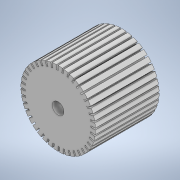
# Autodesk Inventor part: gear(1.5 inch)
Saved by Autodesk Inventor 2022 (Build 260153000, 153)
## iProperties
Created: 2021-07-02
Part Number: gear(1.5 inch)
Material: Generic
Document SubType Name: Modeling
Designer: hp
Density: 1 g/cm^3
Appearance: Default
Author: hp
Autodesk Inventor part; units mm, degrees
ref_plane "YZ Plane" through (0, 0, 0) normal (1, 0, 0) x (0, 1, 0)
ref_plane "XZ Plane" through (0, 0, 0) normal (0, 1, 0) x (-1, 0, 0)
ref_plane "XY Plane" through (0, 0, 0) normal (0, 0, 1) x (1, 0, 0)
sketch "Sketch1" plane through (0, 0, 0) normal (0, 0, 1) x (1, 0, 0)
  circle A0 centre (0, 0) radius 19.05
  dimension "d0" = 38.1
  constraints: 1 centre point, 1 coincident
  measures "d0" diameter of A0
extrude "Extrusion1" add sketch "Sketch1" along normal blind 32.639
sketch "Sketch2" plane through (0, 0, 32.639) normal (0, 0, 1) x (1, 0, 0)
  circle A0 centre (0, 0) radius 19.05 projected
  line L0 (-19.05, 0) -> (-16.815, 0)
  line L1 (-16.815, 0) -> (-16.815, -0.745)
  line L2 (-16.815, -0.745) -> (-19.05, -0.745)
  line L3 (-19.05, -0.745) -> (-19.05, 0)
  line L4 (-18.8155, -2.9801) -> (-16.608, -2.6304)
  line L5 (-16.608, -2.6304) -> (-16.4914, -3.3663)
  line L6 (-16.4914, -3.3663) -> (-18.6989, -3.7159)
  line L7 (-18.6989, -3.7159) -> (-18.8155, -2.9801)
  line L8 (-18.1176, -5.8868) -> (-15.992, -5.1961)
  line L9 (-15.992, -5.1961) -> (-15.7618, -5.9047)
  line L10 (-15.7618, -5.9047) -> (-17.8874, -6.5953)
  line L11 (-17.8874, -6.5953) -> (-18.1176, -5.8868)
  line L12 (-16.9737, -8.6485) -> (-14.9823, -7.6339)
  line L13 (-14.9823, -7.6339) -> (-14.6441, -8.2977)
  line L14 (-14.6441, -8.2977) -> (-16.6355, -9.3123)
  line L15 (-16.6355, -9.3123) -> (-16.9737, -8.6485)
  line L16 (-15.4118, -11.1973) -> (-13.6036, -9.8836)
  line L17 (-13.6036, -9.8836) -> (-13.1657, -10.4863)
  line L18 (-13.1657, -10.4863) -> (-14.9739, -11.8)
  line L19 (-14.9739, -11.8) -> (-15.4118, -11.1973)
  line L20 (-13.4704, -13.4704) -> (-11.89, -11.89)
  line L21 (-11.89, -11.89) -> (-11.3632, -12.4168)
  line L22 (-11.3632, -12.4168) -> (-12.9436, -13.9972)
  line L23 (-12.9436, -13.9972) -> (-13.4704, -13.4704)
  line L24 (-11.1973, -15.4118) -> (-9.8836, -13.6036)
  line L25 (-9.8836, -13.6036) -> (-9.2809, -14.0415)
  line L26 (-9.2809, -14.0415) -> (-10.5946, -15.8497)
  line L27 (-10.5946, -15.8497) -> (-11.1973, -15.4118)
  line L28 (-8.6485, -16.9737) -> (-7.6339, -14.9823)
  line L29 (-7.6339, -14.9823) -> (-6.9701, -15.3205)
  line L30 (-6.9701, -15.3205) -> (-7.9847, -17.3119)
  line L31 (-7.9847, -17.3119) -> (-8.6485, -16.9737)
  line L32 (-5.8868, -18.1176) -> (-5.1961, -15.992)
  line L33 (-5.1961, -15.992) -> (-4.4876, -16.2222)
  line L34 (-4.4876, -16.2222) -> (-5.1782, -18.3478)
  line L35 (-5.1782, -18.3478) -> (-5.8868, -18.1176)
  line L36 (-2.9801, -18.8155) -> (-2.6304, -16.608)
  line L37 (-2.6304, -16.608) -> (-1.8946, -16.7245)
  line L38 (-1.8946, -16.7245) -> (-2.2442, -18.932)
  line L39 (-2.2442, -18.932) -> (-2.9801, -18.8155)
  line L40 (0, -19.05) -> (0, -16.815)
  line L41 (0, -16.815) -> (0.745, -16.815)
  line L42 (0.745, -16.815) -> (0.745, -19.05)
  line L43 (0.745, -19.05) -> (0, -19.05)
  line L44 (2.9801, -18.8155) -> (2.6304, -16.608)
  line L45 (2.6304, -16.608) -> (3.3663, -16.4914)
  line L46 (3.3663, -16.4914) -> (3.7159, -18.6989)
  line L47 (3.7159, -18.6989) -> (2.9801, -18.8155)
  line L48 (5.8868, -18.1176) -> (5.1961, -15.992)
  line L49 (5.1961, -15.992) -> (5.9047, -15.7618)
  line L50 (5.9047, -15.7618) -> (6.5953, -17.8874)
  line L51 (6.5953, -17.8874) -> (5.8868, -18.1176)
  line L52 (8.6485, -16.9737) -> (7.6339, -14.9823)
  line L53 (7.6339, -14.9823) -> (8.2977, -14.6441)
  line L54 (8.2977, -14.6441) -> (9.3123, -16.6355)
  line L55 (9.3123, -16.6355) -> (8.6485, -16.9737)
  line L56 (11.1973, -15.4118) -> (9.8836, -13.6036)
  line L57 (9.8836, -13.6036) -> (10.4863, -13.1657)
  line L58 (10.4863, -13.1657) -> (11.8, -14.9739)
  line L59 (11.8, -14.9739) -> (11.1973, -15.4118)
  line L60 (13.4704, -13.4704) -> (11.89, -11.89)
  line L61 (11.89, -11.89) -> (12.4168, -11.3632)
  line L62 (12.4168, -11.3632) -> (13.9972, -12.9436)
  line L63 (13.9972, -12.9436) -> (13.4704, -13.4704)
  line L64 (15.4118, -11.1973) -> (13.6036, -9.8836)
  line L65 (13.6036, -9.8836) -> (14.0415, -9.2809)
  line L66 (14.0415, -9.2809) -> (15.8497, -10.5946)
  line L67 (15.8497, -10.5946) -> (15.4118, -11.1973)
  line L68 (16.9737, -8.6485) -> (14.9823, -7.6339)
  line L69 (14.9823, -7.6339) -> (15.3205, -6.9701)
  line L70 (15.3205, -6.9701) -> (17.3119, -7.9847)
  line L71 (17.3119, -7.9847) -> (16.9737, -8.6485)
  line L72 (18.1176, -5.8868) -> (15.992, -5.1961)
  line L73 (15.992, -5.1961) -> (16.2222, -4.4876)
  line L74 (16.2222, -4.4876) -> (18.3478, -5.1782)
  line L75 (18.3478, -5.1782) -> (18.1176, -5.8868)
  line L76 (18.8155, -2.9801) -> (16.608, -2.6304)
  line L77 (16.608, -2.6304) -> (16.7245, -1.8946)
  line L78 (16.7245, -1.8946) -> (18.932, -2.2442)
  line L79 (18.932, -2.2442) -> (18.8155, -2.9801)
  line L80 (19.05, 0) -> (16.815, 0)
  line L81 (16.815, 0) -> (16.815, 0.745)
  line L82 (16.815, 0.745) -> (19.05, 0.745)
  line L83 (19.05, 0.745) -> (19.05, 0)
  line L84 (18.8155, 2.9801) -> (16.608, 2.6304)
  line L85 (16.608, 2.6304) -> (16.4914, 3.3663)
  line L86 (16.4914, 3.3663) -> (18.6989, 3.7159)
  line L87 (18.6989, 3.7159) -> (18.8155, 2.9801)
  line L88 (18.1176, 5.8868) -> (15.992, 5.1961)
  line L89 (15.992, 5.1961) -> (15.7618, 5.9047)
  line L90 (15.7618, 5.9047) -> (17.8874, 6.5953)
  line L91 (17.8874, 6.5953) -> (18.1176, 5.8868)
  line L92 (16.9737, 8.6485) -> (14.9823, 7.6339)
  line L93 (14.9823, 7.6339) -> (14.6441, 8.2977)
  line L94 (14.6441, 8.2977) -> (16.6355, 9.3123)
  line L95 (16.6355, 9.3123) -> (16.9737, 8.6485)
  line L96 (15.4118, 11.1973) -> (13.6036, 9.8836)
  line L97 (13.6036, 9.8836) -> (13.1657, 10.4863)
  line L98 (13.1657, 10.4863) -> (14.9739, 11.8)
  line L99 (14.9739, 11.8) -> (15.4118, 11.1973)
  line L100 (13.4704, 13.4704) -> (11.89, 11.89)
  line L101 (11.89, 11.89) -> (11.3632, 12.4168)
  line L102 (11.3632, 12.4168) -> (12.9436, 13.9972)
  line L103 (12.9436, 13.9972) -> (13.4704, 13.4704)
  line L104 (11.1973, 15.4118) -> (9.8836, 13.6036)
  line L105 (9.8836, 13.6036) -> (9.2809, 14.0415)
  line L106 (9.2809, 14.0415) -> (10.5946, 15.8497)
  line L107 (10.5946, 15.8497) -> (11.1973, 15.4118)
  line L108 (8.6485, 16.9737) -> (7.6339, 14.9823)
  line L109 (7.6339, 14.9823) -> (6.9701, 15.3205)
  line L110 (6.9701, 15.3205) -> (7.9847, 17.3119)
  line L111 (7.9847, 17.3119) -> (8.6485, 16.9737)
  line L112 (5.8868, 18.1176) -> (5.1961, 15.992)
  line L113 (5.1961, 15.992) -> (4.4876, 16.2222)
  line L114 (4.4876, 16.2222) -> (5.1782, 18.3478)
  line L115 (5.1782, 18.3478) -> (5.8868, 18.1176)
  line L116 (2.9801, 18.8155) -> (2.6304, 16.608)
  line L117 (2.6304, 16.608) -> (1.8946, 16.7245)
  line L118 (1.8946, 16.7245) -> (2.2442, 18.932)
  line L119 (2.2442, 18.932) -> (2.9801, 18.8155)
  line L120 (0, 19.05) -> (0, 16.815)
  line L121 (0, 16.815) -> (-0.745, 16.815)
  line L122 (-0.745, 16.815) -> (-0.745, 19.05)
  line L123 (-0.745, 19.05) -> (0, 19.05)
  line L124 (-2.9801, 18.8155) -> (-2.6304, 16.608)
  line L125 (-2.6304, 16.608) -> (-3.3663, 16.4914)
  line L126 (-3.3663, 16.4914) -> (-3.7159, 18.6989)
  line L127 (-3.7159, 18.6989) -> (-2.9801, 18.8155)
  line L128 (-5.8868, 18.1176) -> (-5.1961, 15.992)
  line L129 (-5.1961, 15.992) -> (-5.9047, 15.7618)
  line L130 (-5.9047, 15.7618) -> (-6.5953, 17.8874)
  line L131 (-6.5953, 17.8874) -> (-5.8868, 18.1176)
  line L132 (-8.6485, 16.9737) -> (-7.6339, 14.9823)
  line L133 (-7.6339, 14.9823) -> (-8.2977, 14.6441)
  line L134 (-8.2977, 14.6441) -> (-9.3123, 16.6355)
  line L135 (-9.3123, 16.6355) -> (-8.6485, 16.9737)
  line L136 (-11.1973, 15.4118) -> (-9.8836, 13.6036)
  line L137 (-9.8836, 13.6036) -> (-10.4863, 13.1657)
  line L138 (-10.4863, 13.1657) -> (-11.8, 14.9739)
  line L139 (-11.8, 14.9739) -> (-11.1973, 15.4118)
  line L140 (-13.4704, 13.4704) -> (-11.89, 11.89)
  line L141 (-11.89, 11.89) -> (-12.4168, 11.3632)
  line L142 (-12.4168, 11.3632) -> (-13.9972, 12.9436)
  line L143 (-13.9972, 12.9436) -> (-13.4704, 13.4704)
  line L144 (-15.4118, 11.1973) -> (-13.6036, 9.8836)
  line L145 (-13.6036, 9.8836) -> (-14.0415, 9.2809)
  line L146 (-14.0415, 9.2809) -> (-15.8497, 10.5946)
  line L147 (-15.8497, 10.5946) -> (-15.4118, 11.1973)
  line L148 (-16.9737, 8.6485) -> (-14.9823, 7.6339)
  line L149 (-14.9823, 7.6339) -> (-15.3205, 6.9701)
  line L150 (-15.3205, 6.9701) -> (-17.3119, 7.9847)
  line L151 (-17.3119, 7.9847) -> (-16.9737, 8.6485)
  line L152 (-18.1176, 5.8868) -> (-15.992, 5.1961)
  line L153 (-15.992, 5.1961) -> (-16.2222, 4.4876)
  line L154 (-16.2222, 4.4876) -> (-18.3478, 5.1782)
  line L155 (-18.3478, 5.1782) -> (-18.1176, 5.8868)
  line L156 (-18.8155, 2.9801) -> (-16.608, 2.6304)
  line L157 (-16.608, 2.6304) -> (-16.7245, 1.8946)
  line L158 (-16.7245, 1.8946) -> (-18.932, 2.2442)
  line L159 (-18.932, 2.2442) -> (-18.8155, 2.9801)
  dimension "d3" = 2.235
  dimension "d4" = 0.745
  dimension "d7" = 360
  constraints: 320 end point, 2 parallel, 1 horizontal, 1 horizontal alignment, 1 perpendicular, 322 other
  measures "d3" distance of L1.end L2.end
  measures "d4" distance of L0.end L1.end
extrude "Extrusion2" cut sketch "Sketch2" against normal through all contours L80 L81 L82 A0 | A0 L82 L83 | L78 L79 A0 | A0 L76 L77 L78 | L84 L85 L86 A0 | A0 L86 L87 | L74 L75 A0 | A0 L72 L73 L74 | L88 L89 L90 A0 | A0 L90 L91 | L70 L71 A0 | A0 L68 L69 L70 | L92 L93 L94 A0 | A0 L94 L95 | L66 L67 A0 | A0 L64 L65 L66 | L96 L97 L98 A0 | A0 L98 L99 | L62 L63 A0 | A0 L60 L61 L62 | L100 L101 L102 A0 | A0 L102 L103 | L58 L59 A0 | A0 L56 L57 L58 | L104 L105 L106 A0 | A0 L106 L107 | L54 L55 A0 | A0 L52 L53 L54 | L108 L109 L110 A0 | A0 L110 L111 | L50 L51 A0 | A0 L48 L49 L50 | L112 L113 L114 A0 | A0 L114 L115 | L46 L47 A0 | A0 L44 L45 L46 | L116 L117 L118 A0 | A0 L118 L119 | L42 L43 A0 | A0 L40 L41 L42 | L120 L121 L122 A0 | A0 L122 L123 | L38 L39 A0 | A0 L36 L37 L38 | L124 L125 L126 A0 | A0 L126 L127 | L34 L35 A0 | A0 L32 L33 L34 | L128 L129 L130 A0 | A0 L130 L131 | L30 L31 A0 | A0 L28 L29 L30 | L132 L133 L134 A0 | A0 L134 L135 | L26 L27 A0 | A0 L24 L25 L26 | L136 L137 L138 A0 | A0 L138 L139 | L22 L23 A0 | A0 L20 L21 L22 | L140 L141 L142 A0 | A0 L142 L143 | L18 L19 A0 | A0 L16 L17 L18 | L144 L145 L146 A0 | A0 L146 L147 | L14 L15 A0 | A0 L12 L13 L14 | L148 L149 L150 A0 | A0 L150 L151 | L10 L11 A0 | A0 L8 L9 L10 | L152 L153 L154 A0 | A0 L154 L155 | L6 L7 A0 | A0 L4 L5 L6 | L156 L157 L158 A0 | A0 L158 L159 | L2 L3 A0 | A0 L0 L1 L2
sketch "Sketch3" plane through (0, 0, 32.639) normal (0, 0, 1) x (1, 0, 0)
  point P0 (0, 0)
  point P1 (0, 0)
  constraints: 1 coincident
hole "Hole1" at (0, 0, 32.639) direction (0, 0, -1) diameter 6 end through all
body "Solid1"
